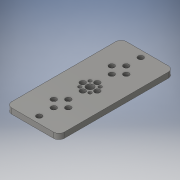
# Autodesk Inventor part: Phone Mount
Saved by Autodesk Inventor 2016 (Build 200138000, 138)
## iProperties
Created: 2015-09-05
Part Number: Phone Mount
Material: ABS Plastic
Document SubType Name: Modeling
Designer: Tim
Density: 1.06 g/cm^3
Appearance: Smooth - Medium Gray
Author: Tim
Autodesk Inventor part; units mm, degrees
ref_plane "YZ Plane" through (0, 0, 0) normal (1, 0, 0) x (0, 1, 0)
ref_plane "XZ Plane" through (0, 0, 0) normal (0, 1, 0) x (-1, 0, 0)
ref_plane "XY Plane" through (0, 0, 0) normal (0, 0, 1) x (1, 0, 0)
sketch "Sketch1" plane through (0, 0, 0) normal (0, 0, 1) x (1, 0, 0)
  line L0 (46.04, 0) -> (0, 0)
  arc A0 (-6, 6) -> (0, 0) centre (0, 6) ccw
  line L1 (-6, 6) -> (-6, 120.62)
  arc A1 (46.04, 0) -> (52.04, 6) centre (46.04, 6) ccw
  line L2 (52.04, 120.62) -> (52.04, 6)
  arc A2 (0, 126.62) -> (-6, 120.62) centre (0, 120.62) ccw
  line L3 (0, 126.62) -> (46.04, 126.62)
  arc A3 (52.04, 120.62) -> (46.04, 126.62) centre (46.04, 120.62) ccw
  circle A4 centre (15.02, 63.31) radius 1.85 projected
  circle A5 centre (17.3631, 68.9669) radius 1.85 projected
  circle A6 centre (23.02, 71.31) radius 1.85 projected
  circle A7 centre (28.6769, 68.9669) radius 1.85 projected
  circle A8 centre (17.3631, 57.6531) radius 1.85 projected
  circle A9 centre (23.02, 55.31) radius 1.85 projected
  circle A10 centre (28.6769, 57.6531) radius 1.85 projected
  circle A11 centre (31.02, 63.31) radius 1.85 projected
  circle A12 centre (23.02, 63.31) radius 4 projected
  circle A13 centre (23.02, 39.31) radius 1.85 projected
  circle A14 centre (23.02, 23.31) radius 1.85 projected
  circle A15 centre (23.02, 7.31) radius 1.85 projected
  circle A16 centre (23.02, 87.31) radius 1.85 projected
  circle A17 centre (23.02, 103.31) radius 1.85 projected
  circle A18 centre (23.02, 119.31) radius 1.85 projected
  circle A19 centre (15.02, 95.31) radius 1.85 projected
  circle A20 centre (31.02, 95.31) radius 1.85 projected
  circle A21 centre (15.02, 31.31) radius 1.85 projected
  circle A22 centre (31.02, 31.31) radius 1.85 projected
  dimension "d18" = 126.62
  dimension "d19" = 58.04
  constraints: 8 end point, 8 point on circle, 4 centre point
  measures "d18" distance between parallel lines of L3 L0
  measures "d19" distance between parallel lines of L1 L2
extrude "Extrusion2" add sketch "Sketch1" along normal mid plane 6
sketch "Sketch3" plane through (0, 0, -3) normal (0, 0, -1) x (-1, 0, 0)
  circle A0 centre (-23.02, 7.31) radius 1.85 projected
  circle A1 centre (-23.02, 23.31) radius 1.85 projected
  circle A2 centre (-31.02, 31.31) radius 1.85 projected
  circle A3 centre (-23.02, 63.31) radius 4 projected
  circle A4 centre (-31.02, 31.31) radius 1.85 projected
  circle A5 centre (-15.02, 31.31) radius 1.85 projected
  circle A6 centre (-31.02, 95.31) radius 1.85 projected
  circle A7 centre (-15.02, 95.31) radius 1.85 projected
  circle A8 centre (-23.02, 119.31) radius 1.85 projected
  circle A9 centre (-23.02, 103.31) radius 1.85 projected
  circle A10 centre (-23.02, 87.31) radius 1.85 projected
  circle A11 centre (-23.02, 7.31) radius 1.85 projected
  circle A12 centre (-23.02, 23.31) radius 1.85 projected
  circle A13 centre (-23.02, 39.31) radius 1.85 projected
  circle A14 centre (-31.02, 63.31) radius 1.85 projected
  circle A15 centre (-28.6769, 57.6531) radius 1.85 projected
  circle A16 centre (-23.02, 55.31) radius 1.85 projected
  circle A17 centre (-17.3631, 57.6531) radius 1.85 projected
  circle A18 centre (-28.6769, 68.9669) radius 1.85 projected
  circle A19 centre (-23.02, 71.31) radius 1.85 projected
  circle A20 centre (-17.3631, 68.9669) radius 1.85 projected
  circle A21 centre (-15.02, 63.31) radius 1.85 projected
  line L0 (-46.04, 0) -> (0, 0) projected
  arc A22 (0, 0) -> (6, 6) centre (0, 6) ccw projected
  line L1 (6, 6) -> (6, 120.62) projected
  arc A23 (6, 120.62) -> (0, 126.62) centre (0, 120.62) ccw projected
  line L2 (0, 126.62) -> (-46.04, 126.62) projected
  arc A24 (-46.04, 126.62) -> (-52.04, 120.62) centre (-46.04, 120.62) ccw projected
  line L3 (-52.04, 120.62) -> (-52.04, 6) projected
  arc A25 (-52.04, 6) -> (-46.04, 0) centre (-46.04, 6) ccw projected
hole "Hole2" at (15.02, 63.31, -3) at (23.02, 71.31, -3) at (31.02, 63.31, -3) at (23.02, 55.31, -3) at (23.02, 87.31, -3) at (15.02, 95.31, -3) at (31.02, 95.31, -3) at (23.02, 103.31, -3) at (23.02, 119.31, -3) at (15.02, 31.31, -3) at (23.02, 39.31, -3) at (23.02, 7.31, -3) at (23.02, 23.31, -3) at (31.02, 31.31, -3) direction (0, 0, 1) diameter 3.7 end through all counterbore diameter 6 counterbore depth 3.5
body "Solid2"
